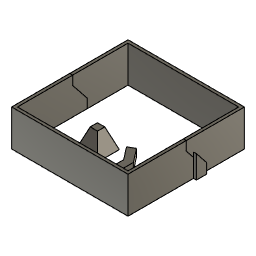
MoldBox (Autodesk Fusion 360 design; units mm, degrees)
Autodesk Fusion 360 part; units mm, degrees
sketch "Top Design" plane through (0, 0, 0) normal (0, 0, 1) x (1, 0, 0)
  circle A0 centre (0, 0) radius 25.5 construction
  line L0 (-38, 38) -> (38, 38)
  line L1 (38, 38) -> (38, -38)
  line L2 (38, -38) -> (-38, -38)
  line L3 (-38, -38) -> (-38, 38)
  line L4 (-38, 38) -> (38, -38) construction
  line L5 (38, 38) -> (-38, -38) construction
  line L6 (-40, 40) -> (40, 40)
  line L7 (40, 40) -> (40, -40)
  line L8 (40, -40) -> (-40, -40)
  line L9 (-40, -40) -> (-40, 40)
  line L10 (-40, 40) -> (40, -40) construction
  line L11 (40, 40) -> (-40, -40) construction
  line L12 (0, 40) -> (0, -40) construction
  line L13 (-2.5, -25.3772) -> (-7.5, -38)
  line L14 (2.5, -25.3772) -> (7.5, -38)
  line L15 (10.3633, -23.2992) -> (17.0935, -32)
  line L16 (17.0935, -32) -> (17.0935, -38)
  line L17 (14.7515, -20.8001) -> (22.0935, -30.2919)
  line L18 (22.0935, -30.2919) -> (22.0935, -38)
  arc A1 (10.3633, -23.2992) -> (14.7515, -20.8001) centre (-1.385, 2.432) ccw
  arc A2 (-2.5, -25.3772) -> (2.5, -25.3772) centre (0, -0.1017) ccw
  dimension "d1" = 51
  dimension "d19" = 76
  dimension "d20" = 80
  dimension "d33" = 15
  dimension "d35" = 2.5
  dimension "d36" = 2.5
  dimension "d37" = 5
  dimension "d38" = 5
  dimension "d44" = 7.5
  dimension "d45" = 12
  dimension "d46" = 6
  dimension "d47" = 11
  dimension "d48" = 25.3988
  constraint coincident A0.centre origin
  constraint horizontal L0
  constraint perpendicular L0 L1
  constraint parallel L0 L2
  constraint parallel L1 L3
  constraint coincident L4 A0.centre
  constraint coincident L5 A0.centre
  constraint equal L0 L3
  constraint horizontal L6
  constraint perpendicular L6 L7
  constraint parallel L6 L8
  constraint parallel L7 L9
  constraint coincident L10 A0.centre
  constraint coincident L11 A0.centre
  constraint equal L6 L9
  constraint midpoint L6 L12.start
  constraint midpoint L8 L12.end
  constraint coincident A0 L13.start
  constraint coincident L2 L13.end
  constraint coincident A0 L14.start
  constraint coincident L2 L14.end
  constraint coincident A0 L15.start
  constraint coincident L2 L16.end
  constraint perpendicular L2 L16
  constraint coincident A0 L17.start
  constraint coincident L2 L18.end
  constraint perpendicular L2 L18
  constraint parallel L15 L17
  constraint tangent A1 A2
  measures "d1" diameter of A0
  measures "d19" distance of L0.start L2.end
  measures "d20" distance of L6.start L8.end
  measures "d33" distance of L13.end L14.end
  measures "d35" distance of L12 L13.start
  measures "d36" distance of L12 L14.start
  measures "d37" distance of L16 L18
  measures "d38" distance of L15 L17
  measures "d44" distance of L12 L13.end
  measures "d45" distance of L17.start L17.end
  measures "d46" distance of L15.end L16.end
  measures "d47" distance of L15.start L15.end
  measures "d48" radius of A2
extrude "Wall Extrude" add sketch "Top Design" along normal blind 25 makes body 1
sketch "Side Box Registration" plane through (-40, 0, 0) normal (-1, 0, 0) x (0, -1, 0)
  line L0 (-40, 0) -> (40, 0)
  line L1 (40, 0) -> (40, 25)
  line L2 (40, 25) -> (-40, 25)
  line L3 (-40, 25) -> (-40, 0)
  line L4 (0, 25) -> (0, 18.75)
  line L5 (0, 18.75) -> (-10, 6.25)
  line L6 (-10, 6.25) -> (-10, 0)
  line L7 (-5, 0) -> (-5, 15.7016)
  line L8 (-5, 15.7016) -> (-12, 6.9516)
  line L9 (-12, 6.9516) -> (-12, 0)
  dimension "d23" = 10
  dimension "d24" = 6.25
  dimension "d25" = 6.25
  dimension "d26" = 2
  dimension "d27" = 2
  dimension "d28" = 5
  constraint midpoint L2 L4.start
  constraint coincident L0 L6.end
  constraint perpendicular L0 L6
  constraint coincident L0 L7.start
  constraint perpendicular L0 L7
  constraint parallel L5 L8
  constraint coincident L0 L9.end
  constraint perpendicular L0 L9
  measures "d23" distance of origin L6.end
  measures "d24" distance of L5.end L6.end
  measures "d25" distance of L4.start L4.end
  measures "d26" distance of L6 L9
  measures "d27" distance of L5 L8
  measures "d28" distance of L4 L7
split "Box Split" by curves path "Side Box Registration" along L4 L5 L6 bodies 1 makes body 2 at (13.3333, -40, 8.3333)
extrude "Registration Extrude" add sketch "Side Box Registration" along normal blind 2 contours L0 L5 L6 L7 L8 L9 | L0 L5 L6 L7 bodies 2
mirror "Mirroring Registration" about plane through (0, 0, 0) normal (1, 0, 0) of "Registration Extrude"
sketch "3D Sprue and Vent" plane through (0, 0, 0) normal (0, 0, 1) x (1, 0, 0)
  line L0 (-2.6333, -3.3517) -> (-17.6333, -3.3517)
  line L1 (-17.6333, -3.3517) -> (-17.6333, -18.3517)
  line L2 (-17.6333, -18.3517) -> (-2.6333, -18.3517)
  line L3 (-2.6333, -18.3517) -> (-2.6333, -3.3517)
  line L4 (-7.6333, -8.3517, 13.5) -> (-12.6333, -8.3517, 13.5)
  line L5 (-12.6333, -8.3517, 13.5) -> (-12.6333, -13.3517, 13.5)
  line L6 (-12.6333, -13.3517, 13.5) -> (-7.6333, -13.3517, 13.5)
  line L7 (-7.6333, -13.3517, 13.5) -> (-7.6333, -8.3517, 13.5)
  line L8 (9.8738, -12.8603) -> (9.8738, -19.8603)
  arc A0 (3.1436, -4.1595) -> (7.5318, -1.6604) centre (-8.6047, 21.5717) ccw
  line L9 (14.8738, -19.8604) -> (9.8738, -19.8604)
  line L10 (9.8738, -19.8603) -> (9.8738, -19.8604)
  line L11 (14.8738, -18.8603) -> (14.8738, -19.8604)
  line L12 (14.8738, -11.1522) -> (14.8738, -18.8603)
  line L13 (3.1436, -4.1595) -> (9.8738, -12.8603)
  line L14 (7.5318, -1.6604) -> (14.8738, -11.1522)
  dimension "d49" = 15
  dimension "d50" = 15
  dimension "d51" = 5
  dimension "d52" = 5
  dimension "d68" = 5
  dimension "d69" = 5
  dimension "d70" = 12
  dimension "d71" = 7
  dimension "d72" = 11
  constraint horizontal L0
  constraint vertical L1
  constraint horizontal L2
  constraint vertical L3
  constraint parallel L13 L14
  constraint perpendicular L9 L10
  measures "d49" distance of L0.start L0.end
  measures "d50" distance of L0.start L2.end
  measures "d68" distance of L8 L12
  measures "d69" distance of L13 L14
  measures "d70" distance of L12.start A0.end
  measures "d71" distance of L8.end L8.start
  measures "d72" distance of A0.start L8.start
sketch "Sprue and Vent Placement" plane through (0, -38, 0) normal (0, 1, 0) x (-1, 0, 0)
  line L0 (-38, 0) -> (38, 0)
  line L1 (38, 0) -> (38, 25)
  line L2 (38, 25) -> (-38, 25)
  line L3 (-38, 25) -> (-38, 0)
  line L4 (-17.0935, 0) -> (-17.0935, 25) construction
  line L5 (-22.0935, 0) -> (-22.0935, 25) construction
  line L6 (-7.5, 0) -> (-7.5, 25) construction
  line L7 (7.5, 0) -> (7.5, 25) construction
  line L8 (-22.0935, 12.5) -> (-17.0935, 12.5) construction
  line L9 (-7.5, 12.5) -> (7.5, 12.5) construction
  line L10 (7.375, 19.875) -> (-7.375, 19.875)
  line L11 (-7.375, 19.875) -> (-7.375, 5.125)
  line L12 (-7.375, 5.125) -> (7.375, 5.125)
  line L13 (7.375, 5.125) -> (7.375, 19.875)
  line L14 (7.375, 19.875) -> (-7.375, 5.125) construction
  line L15 (-7.375, 19.875) -> (7.375, 5.125) construction
  line L16 (-22.0935, 15) -> (-17.0935, 15)
  line L17 (-17.0935, 15) -> (-17.0935, 10)
  line L18 (-17.0935, 10) -> (-22.0935, 10)
  line L19 (-22.0935, 10) -> (-22.0935, 15)
  line L20 (-22.0935, 15) -> (-17.0935, 10) construction
  line L21 (-17.0935, 15) -> (-22.0935, 10) construction
  point P0 (-17.0935, 0)
  point P1 (-22.0935, 0)
  point P2 (-7.5, 0)
  point P3 (7.5, 0)
  point P4 (0, 12.5)
  point P5 (-19.5935, 12.5)
  dimension "d55" = 14.75
  dimension "d56" = 14.75
  dimension "d57" = 5
  dimension "d58" = 5
  constraint coincident P0 L4.start
  constraint coincident L2 L4.end
  constraint perpendicular L2 L4
  constraint coincident P1 L5.start
  constraint coincident L2 L5.end
  constraint perpendicular L2 L5
  constraint coincident P2 L6.start
  constraint coincident L2 L6.end
  constraint perpendicular L2 L6
  constraint coincident P3 L7.start
  constraint coincident L2 L7.end
  constraint perpendicular L2 L7
  constraint midpoint L5 L8.start
  constraint midpoint L7 L9.end
  constraint coincident L4 L8.end
  constraint coincident L6 L9.start
  constraint collinear L8 L9
  constraint horizontal L10
  constraint perpendicular L10 L11
  constraint parallel L10 L12
  constraint parallel L11 L13
  constraint coincident L14 P4
  constraint coincident L15 P4
  constraint midpoint L9 P4
  constraint horizontal L16
  constraint perpendicular L16 L17
  constraint parallel L16 L18
  constraint parallel L17 L19
  constraint coincident L20 P5
  constraint coincident L21 P5
  constraint midpoint L8 P5
  measures "d55" distance of L11.end L12.end
  measures "d56" distance of L10.end L11.end
  measures "d57" distance of L17.end L18.end
  measures "d58" distance of L16.end L17.end
extrude "Placeholder Cut" cut sketch "Sprue and Vent Placement" against normal blind 1 contours L10 L11 L12 L13 | L16 L17 L18 L19 bodies 2
loft "Sprue Loft" add profiles "3D Sprue and Vent", "3D Sprue and Vent" section 1 contours L0 L1 L2 L3 section 2 contours L4 L5 L6 L7 in plane through (0, 0, 13.5) normal (0, 0, 1) separate body makes body 3
extrude "Vent Extrude" add sketch "3D Sprue and Vent" along normal blind 5 separate body contours L8 A0 L9 L11 L12 L13 L14 makes body 4
chamfer "Placeholder Chamfer" distance 1 angle 45 2 edges at (19.5935, -38, 15) (0, -38, 19.875) on bodies 2
named bodies: "Mold Box Left", "Mold Box Right", "Sprue", "Vent"
